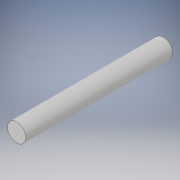
# Autodesk Inventor part: Tube
Saved by Autodesk Inventor 2019 (Build 230136000, 136)
## iProperties
Created: 2019-05-08
Part Number: Tube
Material: Generic
Document SubType Name: Modeling
Designer: riphipps21
Density: 1 g/cm^3
Appearance: Default
Author: riphipps21
Autodesk Inventor part; units mm, degrees
ref_plane "YZ Plane" through (0, 0, 0) normal (1, 0, 0) x (0, 1, 0)
ref_plane "XZ Plane" through (0, 0, 0) normal (0, 1, 0) x (-1, 0, 0)
ref_plane "XY Plane" through (0, 0, 0) normal (0, 0, 1) x (1, 0, 0)
sketch "Sketch1" plane through (0, 0, 0) normal (0, 0, 1) x (1, 0, 0)
  circle A0 centre (0, 0) radius 3.175
  dimension "d1" = 50.8
  constraints: 3 coincident, 1 centre point
extrude "Extrusion1" add sketch "Sketch1" against normal blind 50.8
body "Solid1"
